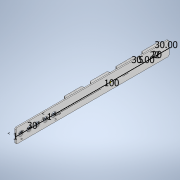
# Autodesk Inventor part: actuator_bone_joint
Saved by Autodesk Inventor 2021 (Build 250183000, 183)
## iProperties
Created: 2021-05-25
Part Number: actuator_bone_joint
Material: Generic
Document SubType Name: Modeling
Designer: Charlie
Density: 1 g/cm^3
Appearance: Default
Author: Charlie
Autodesk Inventor part; units mm, degrees
ref_plane "YZ Plane" through (0, 0, 0) normal (1, 0, 0) x (0, 1, 0)
ref_plane "XZ Plane" through (0, 0, 0) normal (0, 1, 0) x (-1, 0, 0)
ref_plane "XY Plane" through (0, 0, 0) normal (0, 0, 1) x (1, 0, 0)
sketch "Sketch3" plane through (0, 0, 0) normal (0, 1, 0) x (-1, 0, 0)
  line L0 (0.5, -50) -> (-0.5, -50)
  line L1 (-0.5, -50) -> (-0.5, 50)
  line L2 (-0.5, 50) -> (0.5, 50)
  line L3 (0.5, 50) -> (0.5, -50)
  line L4 (0.5, -50) -> (-0.5, 50) construction
  line L5 (-0.5, -50) -> (0.5, 50) construction
  line L6 (0.5, -50) -> (0.5, -30)
  line L7 (0.5, -30) -> (5.5, -30)
  line L8 (5.5, -30) -> (5.5, -50)
  line L9 (5.5, -50) -> (0.5, -50)
  line L10 (0.5, -30) -> (6.2137, -30) construction
  line L11 (0.5, -50) -> (5.5, -47.1132)
  line L12 (0.5, -50) -> (6.2735, -50) construction
  line L13 (0.5, -30) -> (5.5, -32.8868)
  line L14 (0.5, -30) -> (5.6279, -30) construction
  line L15 (0.5, -28) -> (5.5, -25.1132)
  line L16 (5.5, -8) -> (5.5, -28)
  line L17 (0.5, -8) -> (5.5, -10.8868)
  line L18 (0.5, -6) -> (5.5, -3.1132)
  line L19 (5.5, 14) -> (5.5, -6)
  line L20 (0.5, 14) -> (5.5, 11.1132)
  line L21 (0.5, 16) -> (5.5, 18.8868)
  line L22 (5.5, 36) -> (5.5, 16)
  line L23 (0.5, 36) -> (5.5, 33.1132)
  line L24 (-0.5, 50) -> (0.5, 50)
  line L25 (0.5, 50) -> (0.5, 80)
  line L26 (0.5, 80) -> (-0.5, 80)
  line L27 (-0.5, 80) -> (-0.5, 50)
  point P0 (0, 0)
  dimension "d17" = 1
  dimension "d18" = 100
  dimension "d19" = 20
  dimension "d20" = 5
  dimension "d22" = 30
  dimension "d23" = 30
  dimension "d26" = 22
  dimension "d35" = 1
  dimension "d36" = 30
  constraints: 56 end point, 9 point on line, 6 parallel, 5 horizontal, 3 perpendicular, 2 midpoint, 1 equal length, 1 vertical, 27 other
  measures "d17" distance of L1.end L2.end
  measures "d18" distance of L0.end L1.end
  measures "d19" distance of L0.start L6.end
  measures "d20" distance of L6.end L7.end
  measures "d22" angle of L12 L11
  measures "d23" angle of L13 L14
  measures "d26" distance of L0.start L15.start
  measures "d35" distance of L26.end L25.end
  measures "d36" distance of L25.end L24.end
extrude "Extrusion1" add sketch "Sketch3" along normal mid plane 12 contours L0 L1 L2 L3 | L27 L26 L25 L2
extrude "Extrusion2" add sketch "Sketch3" along normal mid plane 6 contours L3 L13 L8 L11 | L3 L17 L16 L15 | L23 L22 L21 L3 | L3 L20 L19 L18
sketch "Sketch4" plane through (-0.5, -6, 80) normal (-1, 0, 0) x (0, 0, 1)
  circle A0 centre (-32, 6) radius 2
  line L0 (-44, 9) -> (-44, 3) projected
  line L1 (-44, 6) -> (0, 6) construction
  line L2 (0, 12) -> (0, 0) construction
  circle A1 centre (-25, 6) radius 2
  circle A2 centre (-18, 6) radius 2
  circle A3 centre (-11, 6) radius 2
  circle A4 centre (-4, 6) radius 2
  point P0 (-80, 6)
  dimension "d37" = 4
  dimension "d38" = 12
  dimension "d41" = 7
  constraints: 5 centre point, 2 end point, 2 midpoint, 1 horizontal, 8 other
  measures "d37" diameter of A0
  measures "d38" distance from line of A0.centre L0
  measures "d41" distance of A0.centre A1.centre
extrude "Extrusion3" cut sketch "Sketch4" against normal blind 6
sketch "Sketch5" plane through (-0.5, 6, 80) normal (0, 0, 1) x (1, 0, 0)
  line L0 (-5, -9) -> (-5, -3) construction
  line L1 (0, -9) -> (0, -3) construction
  line L2 (-5, -9) -> (0, -9) construction
  line L3 (0, -9) -> (0, -3) construction
  line L4 (0, -3) -> (-5, -3) construction
  line L5 (-5, -3) -> (-5, -9) construction
  line L6 (0, -9) -> (-5, -3) construction
  line L7 (-5, -9) -> (0, -3) construction
  line L8 (-2.5, -6) -> (-3.8, -6) construction
  circle A0 centre (-3.8, -6) radius 0.5
  circle A1 centre (-1.85, -7.1258) radius 0.5
  circle A2 centre (-1.85, -4.8742) radius 0.5
  point P0 (0.5, -6)
  dimension "d48" = 6
  dimension "d49" = 1.3
  dimension "d50" = 1
  dimension "d53" = 360
  constraints: 14 end point, 3 centre point, 2 horizontal, 2 parallel, 1 coincident, 1 midpoint, 1 perpendicular, 7 other
  measures "d48" distance of L0.start L0.end
  measures "d49" distance of L8.start L8.end
  measures "d50" diameter of A0
extrude "Extrusion4" cut sketch "Sketch5" against normal blind 150
fillet "Fillet1" radius 1 4 edges at (0, 6, 80) (0, -6, 80) (0, -6, -50) (0, 6, -50)
body "Solid1"
